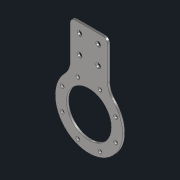
# Autodesk Inventor part: scara-plate8
Saved by Autodesk Inventor 2022 (Build 260153000, 153)
## iProperties
Created: 2021-10-10
Part Number: scara-plate8
Material: 鋼、炭素鋼
Document SubType Name: Sheet Metal
Designer: Yuta Kage
Density: 7.85 g/cm^3
Sheet Metal Rule: Default
Appearance: 半つや出し
Author: Yuta Kage
Autodesk Inventor part; units mm, degrees
ref_plane "YZ Plane" through (0, 0, 0) normal (1, 0, 0) x (0, 1, 0)
ref_plane "XZ Plane" through (0, 0, 0) normal (0, 1, 0) x (-1, 0, 0)
ref_plane "XY Plane" through (0, 0, 0) normal (0, 0, 1) x (1, 0, 0)
sketch "スケッチ1" plane through (0, 0, 0) normal (0, 0, 1) x (1, 0, 0)
  arc A0 (-20, 29.9333) -> (20, 29.9333) centre (0, 0) ccw
  line L0 (-20, -80) -> (20, -80)
  line L1 (20, -80) -> (20, 80)
  line L2 (20, 80) -> (-20, 80)
  line L3 (-20, 80) -> (-20, -80)
  line L4 (-20, -80) -> (20, 80) construction
  line L5 (20, -80) -> (-20, 80) construction
  dimension "d0" = 72
  dimension "d1" = 80
  dimension "d2" = 40
  measures "d0" diameter of A0
  measures "d1" distance from line of point (0, 0) L2
  measures "d2" distance of L1.end L2.end
extrude "プレート1" add sketch "スケッチ1" along normal blind 2.3 contours L3 A0 | L3 L2 L1 A0 | L1 A0
sketch "スケッチ2" plane through (0, 0, 2.3) normal (0, 0, 1) x (1, 0, 0)
  circle A0 centre (0, 0) radius 31
  point P0 (-28.6403, -11.8632)
  point P1 (-11.8632, -28.6403)
  point P2 (11.8632, -28.6403)
  point P3 (28.6403, -11.8632)
  point P4 (28.6403, 11.8632)
  point P5 (11.8632, 28.6403)
  point P6 (-11.8632, 28.6403)
  point P7 (-28.6403, 11.8632)
  dimension "d5" = 62
  dimension "d8" = 360
  dimension "d34" = 0
  constraints: 1 coincident, 12 other
  measures "d34" vertical distance of point (11.863, -28.64) point (-11.863, -28.64)
hole "穴1" at (-28.6403, 11.8632, 2.3) at (-11.8632, 28.6403, 2.3) at (11.8632, 28.6403, 2.3) at (28.6403, 11.8632, 2.3) at (28.6403, -11.8632, 2.3) at (11.8632, -28.6403, 2.3) at (-11.8632, -28.6403, 2.3) at (-28.6403, -11.8632, 2.3) direction (0, 0, -1) diameter 4.3 end through all clearance for "Socket Head Cap Screw" size "M4" standard "Ansi Metric M Profile"
sketch "スケッチ4" plane through (0, 0, 2.3) normal (0, 0, 1) x (1, 0, 0)
  line L0 (10, 50) -> (-10, 50)
  line L1 (-10, 50) -> (-10, 70)
  line L2 (-10, 70) -> (10, 70)
  line L3 (10, 70) -> (10, 50)
  line L4 (10, 50) -> (-10, 70) construction
  line L5 (-10, 50) -> (10, 70) construction
  line L6 (-20, 80) -> (20, 80) projected
  circle A0 centre (0, 0) radius 72.5
  point P0 (0, 60)
  point P1 (0, 60)
  dimension "d21" = 20
  dimension "d22" = 10
  dimension "d33" = 145
  dimension "d38" = 20
  constraints: 12 end point, 3 midpoint, 2 parallel, 1 centre point, 1 coincident, 1 horizontal, 1 perpendicular, 1 vertical alignment
  measures "d21" distance of L1.end L2.end
  measures "d22" distance between parallel lines of L6 L2
  measures "d33" diameter of A0
  measures "d38" distance of L0.end L1.end
hole "穴2" at (-10, 70, 2.3) at (10, 70, 2.3) at (-10, 50, 2.3) at (10, 50, 2.3) direction (0, 0, -1) diameter 5.3 end through all clearance for "Socket Head Cap Screw" size "M5" standard "Ansi Metric M Profile"
fillet "コーナーR2" radius 5 2 edges at (-20, 80, 1.15) (20, 80, 1.15)
sketch "スケッチ5" plane through (0, 0, 2.3) normal (0, 0, 1) x (1, 0, 0)
  circle A0 centre (0, 0) radius 24
  dimension "d35" = 48
  constraints: 1 centre point, 1 coincident
  measures "d35" diameter of A0
extrude "押し出し2" cut sketch "スケッチ5" against normal blind 10
fillet "コーナーR3" radius 20 2 edges at (20, 29.9333, 1.15) (-20, 29.9333, 1.15)
equation "\"d16\" = Thickness"
equation "\"d3\" = Thickness"
equation "\"BendRadius\" = Thickness"
equation "\"BendReliefWidth\" = Thickness"
equation "\"BendReliefDepth\" = 0.5 * Thickness"
equation "\"CornerReliefSize\" = 4 * Thickness"
equation "\"MinimumRemnant\" = 2 * Thickness"
equation "\"TransitionRadius\" = BendRadius"
equation "\"JacobiRadiusSize\" = BendRadius"
equation "\"GapSize\" = Thickness"
equation "\"Thickness\" = 2.3"
